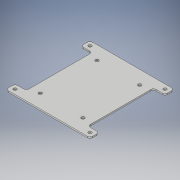
# Autodesk Inventor part: ethernetPlate
Saved by Autodesk Inventor 2018 (Build 220112000, 112)
## iProperties
Created: 2020-02-05
Part Number: ethernetPlate
Material: Generic
Document SubType Name: Modeling
Designer: anirudh.bali
Density: 1 g/cm^3
Appearance: Default
Author: anirudh.bali
Autodesk Inventor part; units mm, degrees
ref_plane "YZ Plane" through (0, 0, 0) normal (1, 0, 0) x (0, 1, 0)
ref_plane "XZ Plane" through (0, 0, 0) normal (0, 1, 0) x (-1, 0, 0)
ref_plane "XY Plane" through (0, 0, 0) normal (0, 0, 1) x (1, 0, 0)
sketch "Sketch1" plane through (0, 0, 0) normal (0, 1, 0) x (-1, 0, 0)
  line L0 (0, 0) -> (93.98, 0)
  line L1 (93.98, -93.98) -> (0, -93.98)
  circle A0 centre (88.9, -5.08) radius 1.75
  circle A1 centre (5.08, -5.08) radius 1.75
  circle A2 centre (5.08, -88.9) radius 1.75
  circle A3 centre (88.9, -88.9) radius 1.75
  circle A4 centre (23.1775, -78.74) radius 1.8
  circle A5 centre (23.1775, -78.74) radius 1.8
  circle A6 centre (70.8025, -78.74) radius 1.8
  circle A7 centre (70.8025, -78.74) radius 1.8
  circle A8 centre (70.8025, -15.24) radius 1.8
  circle A9 centre (70.8025, -15.24) radius 1.8
  circle A10 centre (23.1775, -15.24) radius 1.8
  circle A11 centre (23.1775, -15.24) radius 1.8
  line L2 (93.98, 0) -> (93.98, -10.16)
  line L3 (93.98, -10.16) -> (81.28, -10.16)
  line L4 (93.98, -93.98) -> (93.98, -83.82)
  line L5 (93.98, -83.82) -> (81.28, -83.82)
  line L6 (81.28, -83.82) -> (81.28, -10.16)
  line L7 (0, -10.16) -> (12.7, -10.16)
  line L8 (0, -83.82) -> (12.7, -83.82)
  line L9 (12.7, -83.82) -> (12.7, -10.16)
  line L10 (93.98, 0) -> (93.98, -10.16)
  line L11 (93.98, -83.82) -> (93.98, -93.98)
  line L12 (0, -93.98) -> (0, -83.82)
  line L13 (0, -10.16) -> (0, 0)
  constraints: 28 end point, 12 centre point, 5 parallel, 5 perpendicular, 4 coincident, 1 horizontal
extrude "Extrusion1" add sketch "Sketch1" along normal blind 1.5875
fillet "Fillet1" radius 3.175 12 edges at (0, 0.7937, 0) (0, 0.7937, -10.16) (-12.7, 0.7937, -10.16) (-12.7, 0.7937, -83.82) (0, 0.7937, -83.82) (0, 0.7937, -93.98) (-93.98, 0.7937, 0) (-93.98, 0.7937, -10.16) (-81.28, 0.7937, -10.16) (-81.28, 0.7937, -83.82) (-93.98, 0.7937, -83.82) (-93.98, 0.7937, -93.98)
body "Solid1"
